Autodesk Fusion 360 part; units mm, degrees
note: some values were not read from the file. Chosen so that the rebuilt part matches the saved one: which bodies a step acts on. Set by a fixed rule: which sketch regions a step uses.
(part 2 of 6)
sketch "Sketch66" plane through (0, 0, 40) normal (0, 0, 1) x (-1, 0, 0)
  line L0 (-70.6667, -24.0741) -> (-70.6667, -4)
  line L1 (-70.6667, -4) -> (-88.8889, -4)
  line L2 (-88.8889, -4) -> (-88.8889, 0)
  line L3 (-88.8889, 0) -> (-111.1111, 0)
  line L4 (-111.1111, 0) -> (-111.1111, -4)
  line L5 (-111.1111, -4) -> (-129.3333, -4)
  line L6 (-129.3333, -4) -> (-129.3333, -22.2222)
  line L7 (-129.3333, -22.2222) -> (-137.3333, -22.2222)
  line L8 (-137.3333, -22.2222) -> (-137.3333, -4)
  line L9 (-137.3333, -4) -> (-155.5556, -4)
  line L10 (-155.5556, -4) -> (-155.5556, 0)
  line L11 (-155.5556, 0) -> (-177.7778, 0)
  line L12 (-177.7778, 0) -> (-177.7778, -4)
  line L13 (-177.7778, -4) -> (-196, -4)
  line L14 (-196, -4) -> (-196, -22.2222)
  line L15 (-196, -22.2222) -> (-200, -22.2222)
  line L16 (-200, -22.2222) -> (-200, -44.4444)
  line L17 (-200, -44.4444) -> (-196, -44.4444)
  line L18 (-196, -44.4444) -> (-196, -62.6667)
  line L19 (-196, -62.6667) -> (-177.7778, -62.6667)
  line L20 (-177.7778, -62.6667) -> (-177.7778, -70.6667)
  line L21 (-177.7778, -70.6667) -> (-196, -70.6667)
  line L22 (-196, -70.6667) -> (-196, -88.8889)
  line L23 (-196, -88.8889) -> (-200, -88.8889)
  line L24 (-200, -88.8889) -> (-200, -111.1111)
  line L25 (-200, -111.1111) -> (-196, -111.1111)
  line L26 (-196, -111.1111) -> (-196, -129.3333)
  line L27 (-196, -129.3333) -> (-177.7778, -129.3333)
  line L28 (-177.7778, -129.3333) -> (-177.7778, -137.3333)
  line L29 (-177.7778, -137.3333) -> (-196, -137.3333)
  line L30 (-196, -137.3333) -> (-196, -155.5556)
  line L31 (-196, -155.5556) -> (-200, -155.5556)
  line L32 (-200, -155.5556) -> (-200, -177.7778)
  line L33 (-200, -177.7778) -> (-196, -177.7778)
  line L34 (-196, -177.7778) -> (-196, -196)
  line L35 (-196, -196) -> (-177.7778, -196)
  line L36 (-177.7778, -196) -> (-177.7778, -200)
  line L37 (-177.7778, -200) -> (-155.5556, -200)
  line L38 (-155.5556, -200) -> (-155.5556, -196)
  line L39 (-155.5556, -196) -> (-137.3333, -196)
  line L40 (-137.3333, -196) -> (-137.3333, -177.7778)
  line L41 (-137.3333, -177.7778) -> (-129.3333, -177.7778)
  line L42 (-129.3333, -177.7778) -> (-129.3333, -196)
  line L43 (-129.3333, -196) -> (-111.1111, -196)
  line L44 (-111.1111, -196) -> (-111.1111, -200)
  line L45 (-111.1111, -200) -> (-88.8889, -200)
  line L46 (-88.8889, -200) -> (-88.8889, -196)
  line L47 (-88.8889, -196) -> (-70.6667, -196)
  line L48 (-70.6667, -196) -> (-70.6667, -177.7778)
  line L49 (-70.6667, -177.7778) -> (-62.6667, -177.7778)
  line L50 (-62.6667, -177.7778) -> (-62.6667, -196)
  line L51 (-62.6667, -196) -> (-44.4444, -196)
  line L52 (-44.4444, -196) -> (-44.4444, -200)
  line L53 (-44.4444, -200) -> (-22.2222, -200)
  line L54 (-22.2222, -200) -> (-22.2222, -196)
  line L55 (-22.2222, -196) -> (-4, -196)
  line L56 (-4, -196) -> (-4, -177.7778)
  line L57 (-4, -177.7778) -> (0, -177.7778)
  line L58 (0, -177.7778) -> (0, -155.5556)
  line L59 (0, -155.5556) -> (-4, -155.5556)
  line L60 (-4, -155.5556) -> (-4, -137.3333)
  line L61 (-4, -137.3333) -> (-22.2222, -137.3333)
  line L62 (-22.2222, -137.3333) -> (-22.2222, -129.3333)
  line L63 (-22.2222, -129.3333) -> (-4, -129.3333)
  line L64 (-4, -129.3333) -> (-4, -111.1111)
  line L65 (-4, -111.1111) -> (0, -111.1111)
  line L66 (0, -111.1111) -> (0, -88.8889)
  line L67 (0, -88.8889) -> (-4, -88.8889)
  line L68 (-4, -88.8889) -> (-4, -70.6667)
  line L69 (-4, -70.6667) -> (-22.2222, -70.6667)
  line L70 (-22.2222, -70.6667) -> (-22.2222, -62.6667)
  line L71 (-22.2222, -62.6667) -> (-4, -62.6667)
  line L72 (-4, -62.6667) -> (-4, -44.4444)
  line L73 (-4, -44.4444) -> (0, -44.4444)
  line L74 (0, -44.4444) -> (0, -22.2222)
  line L75 (0, -22.2222) -> (-4, -22.2222)
  line L76 (-4, -22.2222) -> (-4, -4)
  line L77 (-4, -4) -> (-22.2222, -4)
  line L78 (-22.2222, -4) -> (-22.2222, 0)
  line L79 (-22.2222, 0) -> (-44.4444, 0)
  line L80 (-44.4444, 0) -> (-44.4444, -4)
  line L81 (-44.4444, -4) -> (-62.6667, -4)
  line L82 (-62.6667, -4) -> (-62.6667, -24.0741)
  line L83 (-62.6667, -24.0741) -> (-66.1667, -24.0741)
  line L84 (-66.1667, -24.0741) -> (-66.1667, -42.5926)
  line L85 (-66.1667, -42.5926) -> (-62.6667, -42.5926)
  line L86 (-62.6667, -42.5926) -> (-62.6667, -62.6667)
  line L87 (-62.6667, -62.6667) -> (-44.4444, -62.6667)
  line L88 (-44.4444, -62.6667) -> (-44.4444, -70.6667)
  line L89 (-44.4444, -70.6667) -> (-62.6667, -70.6667)
  line L90 (-62.6667, -70.6667) -> (-62.6667, -88.8889)
  line L91 (-62.6667, -88.8889) -> (-70.6667, -88.8889)
  line L92 (-70.6667, -88.8889) -> (-70.6667, -70.6667)
  line L93 (-70.6667, -70.6667) -> (-88.8889, -70.6667)
  line L94 (-88.8889, -70.6667) -> (-88.8889, -62.6667)
  line L95 (-88.8889, -62.6667) -> (-70.6667, -62.6667)
  line L96 (-70.6667, -62.6667) -> (-70.6667, -42.5926)
  line L97 (-70.6667, -42.5926) -> (-67.1667, -42.5926)
  line L98 (-67.1667, -42.5926) -> (-67.1667, -24.0741)
  line L99 (-67.1667, -24.0741) -> (-70.6667, -24.0741)
  line L100 (-129.3333, -70.6667) -> (-129.3333, -88.8889)
  line L101 (-129.3333, -88.8889) -> (-137.3333, -88.8889)
  line L102 (-137.3333, -88.8889) -> (-137.3333, -70.6667)
  line L103 (-137.3333, -70.6667) -> (-155.5556, -70.6667)
  line L104 (-155.5556, -70.6667) -> (-155.5556, -62.6667)
  line L105 (-155.5556, -62.6667) -> (-137.3333, -62.6667)
  line L106 (-137.3333, -62.6667) -> (-137.3333, -44.4444)
  line L107 (-137.3333, -44.4444) -> (-129.3333, -44.4444)
  line L108 (-129.3333, -44.4444) -> (-129.3333, -62.6667)
  line L109 (-129.3333, -62.6667) -> (-111.1111, -62.6667)
  line L110 (-111.1111, -62.6667) -> (-111.1111, -70.6667)
  line L111 (-111.1111, -70.6667) -> (-129.3333, -70.6667)
  line L112 (-129.3333, -137.3333) -> (-129.3333, -155.5556)
  line L113 (-129.3333, -155.5556) -> (-137.3333, -155.5556)
  line L114 (-137.3333, -155.5556) -> (-137.3333, -137.3333)
  line L115 (-137.3333, -137.3333) -> (-155.5556, -137.3333)
  line L116 (-155.5556, -137.3333) -> (-155.5556, -129.3333)
  line L117 (-155.5556, -129.3333) -> (-137.3333, -129.3333)
  line L118 (-137.3333, -129.3333) -> (-137.3333, -111.1111)
  line L119 (-137.3333, -111.1111) -> (-129.3333, -111.1111)
  line L120 (-129.3333, -111.1111) -> (-129.3333, -129.3333)
  line L121 (-129.3333, -129.3333) -> (-111.1111, -129.3333)
  line L122 (-111.1111, -129.3333) -> (-111.1111, -137.3333)
  line L123 (-111.1111, -137.3333) -> (-129.3333, -137.3333)
  line L124 (-62.6667, -137.3333) -> (-62.6667, -155.5556)
  line L125 (-62.6667, -155.5556) -> (-70.6667, -155.5556)
  line L126 (-70.6667, -155.5556) -> (-70.6667, -137.3333)
  line L127 (-70.6667, -137.3333) -> (-88.8889, -137.3333)
  line L128 (-88.8889, -137.3333) -> (-88.8889, -129.3333)
  line L129 (-88.8889, -129.3333) -> (-70.6667, -129.3333)
  line L130 (-70.6667, -129.3333) -> (-70.6667, -111.1111)
  line L131 (-70.6667, -111.1111) -> (-62.6667, -111.1111)
  line L132 (-62.6667, -111.1111) -> (-62.6667, -129.3333)
  line L133 (-62.6667, -129.3333) -> (-44.4444, -129.3333)
  line L134 (-44.4444, -129.3333) -> (-44.4444, -137.3333)
  line L135 (-44.4444, -137.3333) -> (-62.6667, -137.3333)
  line L136 (-22.2222, -70.6667) -> (-24.0741, -70.6667)
  line L137 (-24.0741, -70.6667) -> (-24.0741, -62.6667)
  line L138 (-24.0741, -62.6667) -> (-22.2222, -62.6667)
  line L139 (-22.2222, -62.6667) -> (-22.2222, -70.6667)
  line L140 (-22.2222, -67.1667) -> (-44.4444, -67.1667)
  line L141 (-44.4444, -67.1667) -> (-44.4444, -66.1667)
  line L142 (-44.4444, -66.1667) -> (-22.2222, -66.1667)
  line L143 (-22.2222, -66.1667) -> (-22.2222, -67.1667)
  line L144 (-44.4444, -70.6667) -> (-42.5926, -70.6667)
  line L145 (-42.5926, -70.6667) -> (-42.5926, -62.6667)
  line L146 (-42.5926, -62.6667) -> (-44.4444, -62.6667)
  line L147 (-44.4444, -62.6667) -> (-44.4444, -70.6667)
  line L148 (-4, -44.4444) -> (-0.5, -44.4444)
  line L149 (-0.5, -44.4444) -> (-0.5, -42.5926)
  line L150 (-0.5, -42.5926) -> (-4, -42.5926)
  line L151 (-4, -42.5926) -> (-4, -44.4444)
  line L152 (-4, -22.2222) -> (-0.5, -22.2222)
  line L153 (-0.5, -22.2222) -> (-0.5, -24.0741)
  line L154 (-0.5, -24.0741) -> (-4, -24.0741)
  line L155 (-4, -24.0741) -> (-4, -22.2222)
  line L156 (0, -44.4444) -> (-0.5, -44.4444)
  line L157 (-0.5, -44.4444) -> (-0.5, -22.2222)
  line L158 (-0.5, -22.2222) -> (0, -22.2222)
  line L159 (0, -22.2222) -> (0, -44.4444)
  line L160 (-22.2222, -4) -> (-24.0741, -4)
  line L161 (-24.0741, -4) -> (-24.0741, -0.5)
  line L162 (-24.0741, -0.5) -> (-22.2222, -0.5)
  line L163 (-22.2222, -0.5) -> (-22.2222, -4)
  line L164 (-22.2222, 0) -> (-44.4444, 0)
  line L165 (-44.4444, 0) -> (-44.4444, -0.5)
  line L166 (-44.4444, -0.5) -> (-22.2222, -0.5)
  line L167 (-22.2222, -0.5) -> (-22.2222, 0)
  line L168 (-44.4444, -4) -> (-42.5926, -4)
  line L169 (-42.5926, -4) -> (-42.5926, -0.5)
  line L170 (-42.5926, -0.5) -> (-44.4444, -0.5)
  line L171 (-44.4444, -0.5) -> (-44.4444, -4)
  dimension "d309" = 22.2222
  dimension "d310" = 1.8519
  dimension "d311" = 1.8519
  dimension "d312" = 8
  dimension "d313" = 8
  dimension "d314" = 1
  dimension "d315" = 3.5
  dimension "d319" = 0.5
  dimension "d320" = 3.5
  dimension "d321" = 1.8519
  dimension "d322" = 1.8519
  dimension "d323" = 3.5
  dimension "d324" = 22.2222
  dimension "d327" = 3.5
  dimension "d328" = 0.5
  dimension "d329" = 1.8519
  dimension "d330" = 22.2222
  dimension "d331" = 3.5
  dimension "d332" = 1.8519
  constraint horizontal L136
  constraint vertical L137
  constraint horizontal L138
  constraint vertical L139
  constraint coincident L69.end L70.start
  constraint horizontal L140
  constraint vertical L141
  constraint horizontal L142
  constraint vertical L143
  constraint coincident L70 L140.start
  constraint horizontal L144
  constraint vertical L145
  constraint horizontal L146
  constraint vertical L147
  constraint coincident L88.end L89.start
  constraint horizontal L148
  constraint vertical L149
  constraint horizontal L150
  constraint vertical L151
  constraint coincident L72.end L73.start
  constraint horizontal L152
  constraint vertical L153
  constraint horizontal L154
  constraint vertical L155
  constraint coincident L75.end L76.start
  constraint horizontal L156
  constraint vertical L157
  constraint horizontal L158
  constraint vertical L159
  constraint coincident L73.end L74.start
  constraint horizontal L160
  constraint vertical L161
  constraint horizontal L162
  constraint vertical L163
  constraint coincident L77.end L78.start
  constraint horizontal L164
  constraint vertical L165
  constraint horizontal L166
  constraint vertical L167
  constraint coincident L78.end L79.start
  constraint horizontal L168
  constraint vertical L169
  constraint horizontal L170
  constraint vertical L171
  constraint coincident L80.end L81.start
  measures "d309" distance of L141.end L142.end
  measures "d310" distance of L137.end L70.end
  measures "d311" distance of L145.end L87.end
  measures "d312" distance of L69.end L70.end
  measures "d313" distance of L88.end L87.end
  measures "d314" distance of L140.end L141.end
  measures "d315" distance of L141.end L87.end
  measures "d319" distance of L152.end L74.end
  measures "d320" distance of L75.end L152.end
  measures "d321" distance of L75.end L154.end
  measures "d322" distance of L72.end L150.end
  measures "d323" distance of L149.end L150.end
  measures "d324" distance of L73.end L74.end
  measures "d327" distance of L77.end L162.end
  measures "d328" distance of L78.end L162.end
  measures "d329" distance of L161.end L162.end
  measures "d330" distance of L78.end L79.end
  measures "d331" distance of L80.end L165.end
  measures "d332" distance of L169.end L165.end
extrude "Extrude38" cut sketch "Sketch66" against normal blind 4 contours L88 L140 L144 L145 L147 | L88 L140 L141 L142 L145 L147 | L88 L142 L145 L146 L147 | L137 L140 L142 L145 | L70 L136 L137 L139 L140 | L70 L137 L139 L140 L142 L143 | L70 L137 L138 L139 L142 | L73 L148 L149 L150 L151 L157 | L73 L74 L75 L149 L153 L156 L157 L158 L159 | L80 L166 L168 L169 L170 L171 | L78 L79 L80 L162 L164 L165 L166 L167 L170 | L75 L152 L153 L154 L155 L157 | L78 L160 L161 L162 L163 L166 bodies 13 makes body 14 at (103.7037, 102.3704, 40)
sketch "Sketch67" plane through (0, 0, 0) normal (1, 0, 0) x (0, 1, 0)
sketch "Sketch68" plane through (0, 0, 40) normal (0, 0, 1) x (-1, 0, 0)
  line L0 (-4, -70.6667) -> (-24.0741, -70.6667)
  line L1 (-24.0741, -70.6667) -> (-24.0741, -67.1667)
  line L2 (-24.0741, -67.1667) -> (-42.5926, -67.1667)
  line L3 (-42.5926, -67.1667) -> (-42.5926, -70.6667)
  line L4 (-42.5926, -70.6667) -> (-62.6667, -70.6667)
  line L5 (-62.6667, -70.6667) -> (-62.6667, -88.8889)
  line L6 (-62.6667, -88.8889) -> (-70.6667, -88.8889)
  line L7 (-70.6667, -88.8889) -> (-70.6667, -70.6667)
  line L8 (-70.6667, -70.6667) -> (-88.8889, -70.6667)
  line L9 (-88.8889, -70.6667) -> (-88.8889, -62.6667)
  line L10 (-88.8889, -62.6667) -> (-70.6667, -62.6667)
  line L11 (-70.6667, -62.6667) -> (-70.6667, -42.5926)
  line L12 (-70.6667, -42.5926) -> (-67.1667, -42.5926)
  line L13 (-67.1667, -42.5926) -> (-67.1667, -24.0741)
  line L14 (-67.1667, -24.0741) -> (-70.6667, -24.0741)
  line L15 (-70.6667, -24.0741) -> (-70.6667, -4)
  line L16 (-70.6667, -4) -> (-88.8889, -4)
  line L17 (-88.8889, -4) -> (-88.8889, 0)
  line L18 (-88.8889, 0) -> (-111.1111, 0)
  line L19 (-111.1111, 0) -> (-111.1111, -4)
  line L20 (-111.1111, -4) -> (-129.3333, -4)
  line L21 (-129.3333, -4) -> (-129.3333, -22.2222)
  line L22 (-129.3333, -22.2222) -> (-137.3333, -22.2222)
  line L23 (-137.3333, -22.2222) -> (-137.3333, -4)
  line L24 (-137.3333, -4) -> (-155.5556, -4)
  line L25 (-155.5556, -4) -> (-155.5556, 0)
  line L26 (-155.5556, 0) -> (-177.7778, 0)
  line L27 (-177.7778, 0) -> (-177.7778, -4)
  line L28 (-177.7778, -4) -> (-196, -4)
  line L29 (-196, -4) -> (-196, -22.2222)
  line L30 (-196, -22.2222) -> (-200, -22.2222)
  line L31 (-200, -22.2222) -> (-200, -44.4444)
  line L32 (-200, -44.4444) -> (-196, -44.4444)
  line L33 (-196, -44.4444) -> (-196, -62.6667)
  line L34 (-196, -62.6667) -> (-177.7778, -62.6667)
  line L35 (-177.7778, -62.6667) -> (-177.7778, -70.6667)
  line L36 (-177.7778, -70.6667) -> (-196, -70.6667)
  line L37 (-196, -70.6667) -> (-196, -88.8889)
  line L38 (-196, -88.8889) -> (-200, -88.8889)
  line L39 (-200, -88.8889) -> (-200, -111.1111)
  line L40 (-200, -111.1111) -> (-196, -111.1111)
  line L41 (-196, -111.1111) -> (-196, -129.3333)
  line L42 (-196, -129.3333) -> (-177.7778, -129.3333)
  line L43 (-177.7778, -129.3333) -> (-177.7778, -137.3333)
  line L44 (-177.7778, -137.3333) -> (-196, -137.3333)
  line L45 (-196, -137.3333) -> (-196, -155.5556)
  line L46 (-196, -155.5556) -> (-200, -155.5556)
  line L47 (-200, -155.5556) -> (-200, -177.7778)
  line L48 (-200, -177.7778) -> (-196, -177.7778)
  line L49 (-196, -177.7778) -> (-196, -196)
  line L50 (-196, -196) -> (-177.7778, -196)
  line L51 (-177.7778, -196) -> (-177.7778, -200)
  line L52 (-177.7778, -200) -> (-155.5556, -200)
  line L53 (-155.5556, -200) -> (-155.5556, -196)
  line L54 (-155.5556, -196) -> (-137.3333, -196)
  line L55 (-137.3333, -196) -> (-137.3333, -177.7778)
  line L56 (-137.3333, -177.7778) -> (-129.3333, -177.7778)
  line L57 (-129.3333, -177.7778) -> (-129.3333, -196)
  line L58 (-129.3333, -196) -> (-111.1111, -196)
  line L59 (-111.1111, -196) -> (-111.1111, -200)
  line L60 (-111.1111, -200) -> (-88.8889, -200)
  line L61 (-88.8889, -200) -> (-88.8889, -196)
  line L62 (-88.8889, -196) -> (-70.6667, -196)
  line L63 (-70.6667, -196) -> (-70.6667, -177.7778)
  line L64 (-70.6667, -177.7778) -> (-62.6667, -177.7778)
  line L65 (-62.6667, -177.7778) -> (-62.6667, -196)
  line L66 (-62.6667, -196) -> (-44.4444, -196)
  line L67 (-44.4444, -196) -> (-44.4444, -200)
  line L68 (-44.4444, -200) -> (-22.2222, -200)
  line L69 (-22.2222, -200) -> (-22.2222, -196)
  line L70 (-22.2222, -196) -> (-4, -196)
  line L71 (-4, -196) -> (-4, -177.7778)
  line L72 (-4, -177.7778) -> (0, -177.7778)
  line L73 (0, -177.7778) -> (0, -155.5556)
  line L74 (0, -155.5556) -> (-4, -155.5556)
  line L75 (-4, -155.5556) -> (-4, -137.3333)
  line L76 (-4, -137.3333) -> (-22.2222, -137.3333)
  line L77 (-22.2222, -137.3333) -> (-22.2222, -129.3333)
  line L78 (-22.2222, -129.3333) -> (-4, -129.3333)
  line L79 (-4, -129.3333) -> (-4, -111.1111)
  line L80 (-4, -111.1111) -> (0, -111.1111)
  line L81 (0, -111.1111) -> (0, -88.8889)
  line L82 (0, -88.8889) -> (-4, -88.8889)
  line L83 (-4, -88.8889) -> (-4, -70.6667)
  line L84 (-129.3333, -70.6667) -> (-129.3333, -88.8889)
  line L85 (-129.3333, -88.8889) -> (-137.3333, -88.8889)
  line L86 (-137.3333, -88.8889) -> (-137.3333, -70.6667)
  line L87 (-137.3333, -70.6667) -> (-155.5556, -70.6667)
  line L88 (-155.5556, -70.6667) -> (-155.5556, -62.6667)
  line L89 (-155.5556, -62.6667) -> (-137.3333, -62.6667)
  line L90 (-137.3333, -62.6667) -> (-137.3333, -44.4444)
  line L91 (-137.3333, -44.4444) -> (-129.3333, -44.4444)
  line L92 (-129.3333, -44.4444) -> (-129.3333, -62.6667)
  line L93 (-129.3333, -62.6667) -> (-111.1111, -62.6667)
  line L94 (-111.1111, -62.6667) -> (-111.1111, -70.6667)
  line L95 (-111.1111, -70.6667) -> (-129.3333, -70.6667)
  line L96 (-129.3333, -137.3333) -> (-129.3333, -155.5556)
  line L97 (-129.3333, -155.5556) -> (-137.3333, -155.5556)
  line L98 (-137.3333, -155.5556) -> (-137.3333, -137.3333)
  line L99 (-137.3333, -137.3333) -> (-155.5556, -137.3333)
  line L100 (-155.5556, -137.3333) -> (-155.5556, -129.3333)
  line L101 (-155.5556, -129.3333) -> (-137.3333, -129.3333)
  line L102 (-137.3333, -129.3333) -> (-137.3333, -111.1111)
  line L103 (-137.3333, -111.1111) -> (-129.3333, -111.1111)
  line L104 (-129.3333, -111.1111) -> (-129.3333, -129.3333)
  line L105 (-129.3333, -129.3333) -> (-111.1111, -129.3333)
  line L106 (-111.1111, -129.3333) -> (-111.1111, -137.3333)
  line L107 (-111.1111, -137.3333) -> (-129.3333, -137.3333)
  line L108 (-62.6667, -137.3333) -> (-62.6667, -155.5556)
  line L109 (-62.6667, -155.5556) -> (-70.6667, -155.5556)
  line L110 (-70.6667, -155.5556) -> (-70.6667, -137.3333)
  line L111 (-70.6667, -137.3333) -> (-88.8889, -137.3333)
  line L112 (-88.8889, -137.3333) -> (-88.8889, -129.3333)
  line L113 (-88.8889, -129.3333) -> (-70.6667, -129.3333)
  line L114 (-70.6667, -129.3333) -> (-70.6667, -111.1111)
  line L115 (-70.6667, -111.1111) -> (-62.6667, -111.1111)
  line L116 (-62.6667, -111.1111) -> (-62.6667, -129.3333)
  line L117 (-62.6667, -129.3333) -> (-44.4444, -129.3333)
  line L118 (-44.4444, -129.3333) -> (-44.4444, -137.3333)
  line L119 (-44.4444, -137.3333) -> (-62.6667, -137.3333)
  line L120 (-88.8889, -4) -> (-90.7407, -4)
  line L121 (-90.7407, -4) -> (-90.7407, -0.5)
  line L122 (-90.7407, -0.5) -> (-88.8889, -0.5)
  line L123 (-88.8889, -0.5) -> (-88.8889, -4)
  line L124 (-88.8889, 0) -> (-111.1111, 0)
  line L125 (-111.1111, 0) -> (-111.1111, -0.5)
  line L126 (-111.1111, -0.5) -> (-88.8889, -0.5)
  line L127 (-88.8889, -0.5) -> (-88.8889, 0)
  line L128 (-111.1111, -4) -> (-109.2593, -4)
  line L129 (-109.2593, -4) -> (-109.2593, -0.5)
  line L130 (-109.2593, -0.5) -> (-111.1111, -0.5)
  line L131 (-111.1111, -0.5) -> (-111.1111, -4)
  line L132 (-129.3333, -44.4444) -> (-137.3333, -44.4444)
  line L133 (-137.3333, -44.4444) -> (-137.3333, -42.5926)
  line L134 (-137.3333, -42.5926) -> (-129.3333, -42.5926)
  line L135 (-129.3333, -42.5926) -> (-129.3333, -44.4444)
  line L136 (-132.8333, -44.4444) -> (-133.8333, -44.4444)
  line L137 (-133.8333, -44.4444) -> (-133.8333, -22.2222)
  line L138 (-133.8333, -22.2222) -> (-132.8333, -22.2222)
  line L139 (-132.8333, -22.2222) -> (-132.8333, -44.4444)
  line L140 (-129.3333, -22.2222) -> (-137.3333, -22.2222)
  line L141 (-137.3333, -22.2222) -> (-137.3333, -24.0741)
  line L142 (-137.3333, -24.0741) -> (-129.3333, -24.0741)
  line L143 (-129.3333, -24.0741) -> (-129.3333, -22.2222)
  line L144 (-88.8889, -70.6667) -> (-90.7407, -70.6667)
  line L145 (-90.7407, -70.6667) -> (-90.7407, -62.6667)
  line L146 (-90.7407, -62.6667) -> (-88.8889, -62.6667)
  line L147 (-88.8889, -62.6667) -> (-88.8889, -70.6667)
  line L148 (-111.1111, -70.6667) -> (-109.2593, -70.6667)
  line L149 (-109.2593, -70.6667) -> (-109.2593, -62.6667)
  line L150 (-109.2593, -62.6667) -> (-111.1111, -62.6667)
  line L151 (-111.1111, -62.6667) -> (-111.1111, -70.6667)
  line L152 (-88.8889, -67.1667) -> (-111.1111, -67.1667)
  line L153 (-111.1111, -67.1667) -> (-111.1111, -66.1667)
  line L154 (-111.1111, -66.1667) -> (-88.8889, -66.1667)
  line L155 (-88.8889, -66.1667) -> (-88.8889, -67.1667)
  dimension "d335" = 0.5
  dimension "d337" = 3.5
  dimension "d338" = 1.8519
  dimension "d339" = 22.2222
  dimension "d340" = 1.8519
  dimension "d341" = 3.5
  dimension "d342" = 1.8519
  dimension "d343" = 8
  dimension "d344" = 22.2222
  dimension "d345" = 1
  dimension "d346" = 3.5
  dimension "d347" = 1.8519
  dimension "d348" = 8
  dimension "d349" = 1.8519
  dimension "d350" = 8
  dimension "d351" = 1
  dimension "d352" = 22.2222
  dimension "d353" = 3.5
  dimension "d354" = 1.8519
  dimension "d355" = 8
  dimension "d356" = 3.5
  constraint horizontal L120
  constraint vertical L121
  constraint horizontal L122
  constraint vertical L123
  constraint coincident L16.end L17.start
  constraint horizontal L124
  constraint vertical L125
  constraint horizontal L126
  constraint vertical L127
  constraint coincident L17.end L18.start
  constraint horizontal L128
  constraint vertical L129
  constraint horizontal L130
  constraint vertical L131
  constraint coincident L19.end L20.start
  constraint horizontal L132
  constraint vertical L133
  constraint horizontal L134
  constraint vertical L135
  constraint coincident L91.end L92.start
  constraint horizontal L136
  constraint vertical L137
  constraint horizontal L138
  constraint vertical L139
  constraint coincident L91 L136.start
  constraint horizontal L140
  constraint vertical L141
  constraint horizontal L142
  constraint vertical L143
  constraint coincident L21.end L22.start
  constraint horizontal L144
  constraint vertical L145
  constraint horizontal L146
  constraint vertical L147
  constraint coincident L8.end L9.start
  constraint horizontal L148
  constraint vertical L149
  constraint horizontal L150
  constraint vertical L151
  constraint coincident L94.end L95.start
  constraint horizontal L152
  constraint vertical L153
  constraint horizontal L154
  constraint vertical L155
  constraint coincident L147 L152.start
  measures "d335" distance of L17.end L122.end
  measures "d337" distance of L16.end L122.end
  measures "d338" distance of L121.end L122.end
  measures "d339" distance of L17.end L18.end
  measures "d340" distance of L129.end L125.end
  measures "d341" distance of L19.end L125.end
  measures "d342" distance of L22.end L141.end
  measures "d343" distance of L21.end L22.end
  measures "d344" distance of L136.end L137.end
  measures "d345" distance of L137.end L138.end
  measures "d346" distance of L22.end L137.end
  measures "d347" distance of L90.end L133.end
  measures "d348" distance of L133.end L134.end
  measures "d349" distance of L149.end L93.end
  measures "d350" distance of L94.end L93.end
  measures "d351" distance of L152.end L153.end
  measures "d352" distance of L153.end L154.end
  measures "d353" distance of L93.end L153.end
  measures "d354" distance of L8.end L144.end
  measures "d355" distance of L144.end L145.end
  measures "d356" distance of L9.end L154.end
extrude "Extrude39" cut sketch "Sketch68" against normal blind 4 contours L9 L144 L145 L147 L152 | L9 L145 L147 L152 L154 L155 | L9 L145 L146 L147 L154 | L145 L149 L152 L154 | L94 L149 L151 L152 L153 L154 | L94 L148 L149 L151 L152 | L94 L149 L150 L151 L154 | L91 L132 L134 L135 L139 | L91 L132 L134 L136 L137 L139 | L17 L120 L121 L122 L123 L126 | L91 L132 L133 L134 L137 | L134 L137 L139 L142 | L17 L18 L19 L122 L124 L125 L126 L127 L130 | L22 L137 L138 L139 L140 L142 | L22 L139 L140 L142 L143 | L22 L137 L140 L141 L142 | L19 L126 L128 L129 L130 L131 bodies 14 makes body 15 at (103.7037, 169.037, 40)
sketch "Sketch71" plane through (0, 0, 40) normal (0, 0, 1) x (-1, 0, 0)
  line L0 (-109.2593, -70.6667) -> (-129.3333, -70.6667)
  line L1 (-129.3333, -70.6667) -> (-129.3333, -88.8889)
  line L2 (-129.3333, -88.8889) -> (-137.3333, -88.8889)
  line L3 (-137.3333, -88.8889) -> (-137.3333, -70.6667)
  line L4 (-137.3333, -70.6667) -> (-155.5556, -70.6667)
  line L5 (-155.5556, -70.6667) -> (-155.5556, -62.6667)
  line L6 (-155.5556, -62.6667) -> (-137.3333, -62.6667)
  line L7 (-137.3333, -62.6667) -> (-137.3333, -42.5926)
  line L8 (-137.3333, -42.5926) -> (-133.8333, -42.5926)
  line L9 (-133.8333, -42.5926) -> (-133.8333, -24.0741)
  line L10 (-133.8333, -24.0741) -> (-137.3333, -24.0741)
  line L11 (-137.3333, -24.0741) -> (-137.3333, -4)
  line L12 (-137.3333, -4) -> (-155.5556, -4)
  line L13 (-155.5556, -4) -> (-155.5556, 0)
  line L14 (-155.5556, 0) -> (-177.7778, 0)
  line L15 (-177.7778, 0) -> (-177.7778, -4)
  line L16 (-177.7778, -4) -> (-196, -4)
  line L17 (-196, -4) -> (-196, -22.2222)
  line L18 (-196, -22.2222) -> (-200, -22.2222)
  line L19 (-200, -22.2222) -> (-200, -44.4444)
  line L20 (-200, -44.4444) -> (-196, -44.4444)
  line L21 (-196, -44.4444) -> (-196, -62.6667)
  line L22 (-196, -62.6667) -> (-177.7778, -62.6667)
  line L23 (-177.7778, -62.6667) -> (-177.7778, -70.6667)
  line L24 (-177.7778, -70.6667) -> (-196, -70.6667)
  line L25 (-196, -70.6667) -> (-196, -88.8889)
  line L26 (-196, -88.8889) -> (-200, -88.8889)
  line L27 (-200, -88.8889) -> (-200, -111.1111)
  line L28 (-200, -111.1111) -> (-196, -111.1111)
  line L29 (-196, -111.1111) -> (-196, -129.3333)
  line L30 (-196, -129.3333) -> (-177.7778, -129.3333)
  line L31 (-177.7778, -129.3333) -> (-177.7778, -137.3333)
  line L32 (-177.7778, -137.3333) -> (-196, -137.3333)
  line L33 (-196, -137.3333) -> (-196, -155.5556)
  line L34 (-196, -155.5556) -> (-200, -155.5556)
  line L35 (-200, -155.5556) -> (-200, -177.7778)
  line L36 (-200, -177.7778) -> (-196, -177.7778)
  line L37 (-196, -177.7778) -> (-196, -196)
  line L38 (-196, -196) -> (-177.7778, -196)
  line L39 (-177.7778, -196) -> (-177.7778, -200)
  line L40 (-177.7778, -200) -> (-155.5556, -200)
  line L41 (-155.5556, -200) -> (-155.5556, -196)
  line L42 (-155.5556, -196) -> (-137.3333, -196)
  line L43 (-137.3333, -196) -> (-137.3333, -177.7778)
  line L44 (-137.3333, -177.7778) -> (-129.3333, -177.7778)
  line L45 (-129.3333, -177.7778) -> (-129.3333, -196)
  line L46 (-129.3333, -196) -> (-111.1111, -196)
  line L47 (-111.1111, -196) -> (-111.1111, -200)
  line L48 (-111.1111, -200) -> (-88.8889, -200)
  line L49 (-88.8889, -200) -> (-88.8889, -196)
  line L50 (-88.8889, -196) -> (-70.6667, -196)
  line L51 (-70.6667, -196) -> (-70.6667, -177.7778)
  line L52 (-70.6667, -177.7778) -> (-62.6667, -177.7778)
  line L53 (-62.6667, -177.7778) -> (-62.6667, -196)
  line L54 (-62.6667, -196) -> (-44.4444, -196)
  line L55 (-44.4444, -196) -> (-44.4444, -200)
  line L56 (-44.4444, -200) -> (-22.2222, -200)
  line L57 (-22.2222, -200) -> (-22.2222, -196)
  line L58 (-22.2222, -196) -> (-4, -196)
  line L59 (-4, -196) -> (-4, -177.7778)
  line L60 (-4, -177.7778) -> (0, -177.7778)
  line L61 (0, -177.7778) -> (0, -155.5556)
  line L62 (0, -155.5556) -> (-4, -155.5556)
  line L63 (-4, -155.5556) -> (-4, -137.3333)
  line L64 (-4, -137.3333) -> (-22.2222, -137.3333)
  line L65 (-22.2222, -137.3333) -> (-22.2222, -129.3333)
  line L66 (-22.2222, -129.3333) -> (-4, -129.3333)
  line L67 (-4, -129.3333) -> (-4, -111.1111)
  line L68 (-4, -111.1111) -> (0, -111.1111)
  line L69 (0, -111.1111) -> (0, -88.8889)
  line L70 (0, -88.8889) -> (-4, -88.8889)
  line L71 (-4, -88.8889) -> (-4, -70.6667)
  line L72 (-4, -70.6667) -> (-24.0741, -70.6667)
  line L73 (-24.0741, -70.6667) -> (-24.0741, -67.1667)
  line L74 (-24.0741, -67.1667) -> (-42.5926, -67.1667)
  line L75 (-42.5926, -67.1667) -> (-42.5926, -70.6667)
  line L76 (-42.5926, -70.6667) -> (-62.6667, -70.6667)
  line L77 (-62.6667, -70.6667) -> (-62.6667, -88.8889)
  line L78 (-62.6667, -88.8889) -> (-70.6667, -88.8889)
  line L79 (-70.6667, -88.8889) -> (-70.6667, -70.6667)
  line L80 (-70.6667, -70.6667) -> (-90.7407, -70.6667)
  line L81 (-90.7407, -70.6667) -> (-90.7407, -67.1667)
  line L82 (-90.7407, -67.1667) -> (-109.2593, -67.1667)
  line L83 (-109.2593, -67.1667) -> (-109.2593, -70.6667)
  line L84 (-129.3333, -137.3333) -> (-129.3333, -155.5556)
  line L85 (-129.3333, -155.5556) -> (-137.3333, -155.5556)
  line L86 (-137.3333, -155.5556) -> (-137.3333, -137.3333)
  line L87 (-137.3333, -137.3333) -> (-155.5556, -137.3333)
  line L88 (-155.5556, -137.3333) -> (-155.5556, -129.3333)
  line L89 (-155.5556, -129.3333) -> (-137.3333, -129.3333)
  line L90 (-137.3333, -129.3333) -> (-137.3333, -111.1111)
  line L91 (-137.3333, -111.1111) -> (-129.3333, -111.1111)
  line L92 (-129.3333, -111.1111) -> (-129.3333, -129.3333)
  line L93 (-129.3333, -129.3333) -> (-111.1111, -129.3333)
  line L94 (-111.1111, -129.3333) -> (-111.1111, -137.3333)
  line L95 (-111.1111, -137.3333) -> (-129.3333, -137.3333)
  line L96 (-62.6667, -137.3333) -> (-62.6667, -155.5556)
  line L97 (-62.6667, -155.5556) -> (-70.6667, -155.5556)
  line L98 (-70.6667, -155.5556) -> (-70.6667, -137.3333)
  line L99 (-70.6667, -137.3333) -> (-88.8889, -137.3333)
  line L100 (-88.8889, -137.3333) -> (-88.8889, -129.3333)
  line L101 (-88.8889, -129.3333) -> (-70.6667, -129.3333)
  line L102 (-70.6667, -129.3333) -> (-70.6667, -111.1111)
  line L103 (-70.6667, -111.1111) -> (-62.6667, -111.1111)
  line L104 (-62.6667, -111.1111) -> (-62.6667, -129.3333)
  line L105 (-62.6667, -129.3333) -> (-44.4444, -129.3333)
  line L106 (-44.4444, -129.3333) -> (-44.4444, -137.3333)
  line L107 (-44.4444, -137.3333) -> (-62.6667, -137.3333)
  line L108 (-155.5556, -4) -> (-157.4074, -4)
  line L109 (-157.4074, -4) -> (-157.4074, -0.5)
  line L110 (-157.4074, -0.5) -> (-155.5556, -0.5)
  line L111 (-155.5556, -0.5) -> (-155.5556, -4)
  line L112 (-177.7778, -4) -> (-175.9259, -4)
  line L113 (-175.9259, -4) -> (-175.9259, -0.5)
  line L114 (-175.9259, -0.5) -> (-177.7778, -0.5)
  line L115 (-177.7778, -0.5) -> (-177.7778, -4)
  line L116 (-155.5556, 0) -> (-177.7778, 0)
  line L117 (-177.7778, 0) -> (-177.7778, -0.5)
  line L118 (-177.7778, -0.5) -> (-155.5556, -0.5)
  line L119 (-155.5556, -0.5) -> (-155.5556, 0)
  line L120 (-196, -44.4444) -> (-199.5, -44.4444)
  line L121 (-199.5, -44.4444) -> (-199.5, -42.5926)
  line L122 (-199.5, -42.5926) -> (-196, -42.5926)
  line L123 (-196, -42.5926) -> (-196, -44.4444)
  line L124 (-196, -22.2222) -> (-199.5, -22.2222)
  line L125 (-199.5, -22.2222) -> (-199.5, -24.0741)
  line L126 (-199.5, -24.0741) -> (-196, -24.0741)
  line L127 (-196, -24.0741) -> (-196, -22.2222)
  line L128 (-200, -22.2222) -> (-199.5, -22.2222)
  line L129 (-199.5, -22.2222) -> (-199.5, -44.4444)
  line L130 (-199.5, -44.4444) -> (-200, -44.4444)
  line L131 (-200, -44.4444) -> (-200, -22.2222)
  line L132 (-155.5556, -62.6667) -> (-157.4074, -62.6667)
  line L133 (-157.4074, -62.6667) -> (-157.4074, -70.6667)
  line L134 (-157.4074, -70.6667) -> (-155.5556, -70.6667)
  line L135 (-155.5556, -70.6667) -> (-155.5556, -62.6667)
  line L136 (-177.7778, -62.6667) -> (-175.9259, -62.6667)
  line L137 (-175.9259, -62.6667) -> (-175.9259, -70.6667)
  line L138 (-175.9259, -70.6667) -> (-177.7778, -70.6667)
  line L139 (-177.7778, -70.6667) -> (-177.7778, -62.6667)
  line L140 (-155.5556, -67.1667) -> (-177.7778, -67.1667)
  line L141 (-177.7778, -67.1667) -> (-177.7778, -66.1667)
  line L142 (-177.7778, -66.1667) -> (-155.5556, -66.1667)
  line L143 (-155.5556, -66.1667) -> (-155.5556, -67.1667)
  dimension "d363" = 3.5
  dimension "d364" = 0.5
  dimension "d365" = 22.2222
  dimension "d366" = 1.8519
  dimension "d367" = 1.8519
  dimension "d368" = 3.5
  dimension "d369" = 3.5
  dimension "d370" = 0.5
  dimension "d371" = 1.8519
  dimension "d372" = 22.2222
  dimension "d373" = 3.5
  dimension "d374" = 1.8519
  dimension "d375" = 1.8519
  dimension "d376" = 1.8519
  dimension "d377" = 8
  dimension "d378" = 8
  dimension "d379" = 1
  dimension "d380" = 3.5
  dimension "d381" = 22.2222
  constraint horizontal L108
  constraint vertical L109
  constraint horizontal L110
  constraint vertical L111
  constraint coincident L12.end L13.start
  constraint horizontal L112
  constraint vertical L113
  constraint horizontal L114
  constraint vertical L115
  constraint coincident L15.end L16.start
  constraint horizontal L116
  constraint vertical L117
  constraint horizontal L118
  constraint vertical L119
  constraint coincident L13.end L14.start
  constraint horizontal L120
  constraint vertical L121
  constraint horizontal L122
  constraint vertical L123
  constraint coincident L20.end L21.start
  constraint horizontal L124
  constraint vertical L125
  constraint horizontal L126
  constraint vertical L127
  constraint coincident L17.end L18.start
  constraint horizontal L128
  constraint vertical L129
  constraint horizontal L130
  constraint vertical L131
  constraint coincident L18.end L19.start
  constraint horizontal L132
  constraint vertical L133
  constraint horizontal L134
  constraint vertical L135
  constraint coincident L5.end L6.start
  constraint horizontal L136
  constraint vertical L137
  constraint horizontal L138
  constraint vertical L139
  constraint coincident L22.end L23.start
  constraint horizontal L140
  constraint vertical L141
  constraint horizontal L142
  constraint vertical L143
  constraint coincident L135 L140.start
  measures "d363" distance of L15.end L114.end
  measures "d364" distance of L14.end L114.end
  measures "d365" distance of L13.end L14.end
  measures "d366" distance of L109.end L110.end
  measures "d367" distance of L15.end L112.end
  measures "d368" distance of L12.end L110.end
  measures "d369" distance of L17.end L124.end
  measures "d370" distance of L18.end L124.end
  measures "d371" distance of L17.end L126.end
  measures "d372" distance of L18.end L19.end
  measures "d373" distance of L20.end L120.end
  measures "d374" distance of L20.end L122.end
  measures "d375" distance of L5.end L132.end
  measures "d376" distance of L22.end L136.end
  measures "d377" distance of L136.end L137.end
  measures "d378" distance of L5.end L4.end
  measures "d379" distance of L140.end L141.end
  measures "d380" distance of L4.end L140.start
  measures "d381" distance of L141.end L142.end
extrude "Extrude40" cut sketch "Sketch71" against normal blind 4 contours L5 L133 L134 L135 L140 | L5 L133 L135 L140 L142 L143 | L5 L132 L133 L135 L142 | L133 L137 L140 L142 | L23 L137 L139 L140 L141 L142 | L23 L137 L138 L139 L140 | L23 L136 L137 L139 L142 | L20 L120 L121 L122 L123 L129 | L18 L19 L20 L121 L125 L128 L129 L130 L131 | L13 L108 L109 L110 L111 L118 | L13 L14 L15 L110 L114 L116 L117 L118 L119 | L18 L124 L125 L126 L127 L129 | L15 L112 L113 L114 L115 L118 bodies 15 makes body 16 at (96.2963, 169.037, 40)
sketch "Sketch72" plane through (0, 0, 40) normal (0, 0, 1) x (-1, 0, 0)
  line L0 (-175.9259, -70.6667) -> (-196, -70.6667)
  line L1 (-196, -70.6667) -> (-196, -88.8889)
  line L2 (-196, -88.8889) -> (-200, -88.8889)
  line L3 (-200, -88.8889) -> (-200, -111.1111)
  line L4 (-200, -111.1111) -> (-196, -111.1111)
  line L5 (-196, -111.1111) -> (-196, -129.3333)
  line L6 (-196, -129.3333) -> (-177.7778, -129.3333)
  line L7 (-177.7778, -129.3333) -> (-177.7778, -137.3333)
  line L8 (-177.7778, -137.3333) -> (-196, -137.3333)
  line L9 (-196, -137.3333) -> (-196, -155.5556)
  line L10 (-196, -155.5556) -> (-200, -155.5556)
  line L11 (-200, -155.5556) -> (-200, -177.7778)
  line L12 (-200, -177.7778) -> (-196, -177.7778)
  line L13 (-196, -177.7778) -> (-196, -196)
  line L14 (-196, -196) -> (-177.7778, -196)
  line L15 (-177.7778, -196) -> (-177.7778, -200)
  line L16 (-177.7778, -200) -> (-155.5556, -200)
  line L17 (-155.5556, -200) -> (-155.5556, -196)
  line L18 (-155.5556, -196) -> (-137.3333, -196)
  line L19 (-137.3333, -196) -> (-137.3333, -177.7778)
  line L20 (-137.3333, -177.7778) -> (-129.3333, -177.7778)
  line L21 (-129.3333, -177.7778) -> (-129.3333, -196)
  line L22 (-129.3333, -196) -> (-111.1111, -196)
  line L23 (-111.1111, -196) -> (-111.1111, -200)
  line L24 (-111.1111, -200) -> (-88.8889, -200)
  line L25 (-88.8889, -200) -> (-88.8889, -196)
  line L26 (-88.8889, -196) -> (-70.6667, -196)
  line L27 (-70.6667, -196) -> (-70.6667, -177.7778)
  line L28 (-70.6667, -177.7778) -> (-62.6667, -177.7778)
  line L29 (-62.6667, -177.7778) -> (-62.6667, -196)
  line L30 (-62.6667, -196) -> (-44.4444, -196)
  line L31 (-44.4444, -196) -> (-44.4444, -200)
  line L32 (-44.4444, -200) -> (-22.2222, -200)
  line L33 (-22.2222, -200) -> (-22.2222, -196)
  line L34 (-22.2222, -196) -> (-4, -196)
  line L35 (-4, -196) -> (-4, -177.7778)
  line L36 (-4, -177.7778) -> (0, -177.7778)
  line L37 (0, -177.7778) -> (0, -155.5556)
  line L38 (0, -155.5556) -> (-4, -155.5556)
  line L39 (-4, -155.5556) -> (-4, -137.3333)
  line L40 (-4, -137.3333) -> (-22.2222, -137.3333)
  line L41 (-22.2222, -137.3333) -> (-22.2222, -129.3333)
  line L42 (-22.2222, -129.3333) -> (-4, -129.3333)
  line L43 (-4, -129.3333) -> (-4, -111.1111)
  line L44 (-4, -111.1111) -> (0, -111.1111)
  line L45 (0, -111.1111) -> (0, -88.8889)
  line L46 (0, -88.8889) -> (-4, -88.8889)
  line L47 (-4, -88.8889) -> (-4, -70.6667)
  line L48 (-4, -70.6667) -> (-24.0741, -70.6667)
  line L49 (-24.0741, -70.6667) -> (-24.0741, -67.1667)
  line L50 (-24.0741, -67.1667) -> (-42.5926, -67.1667)
  line L51 (-42.5926, -67.1667) -> (-42.5926, -70.6667)
  line L52 (-42.5926, -70.6667) -> (-62.6667, -70.6667)
  line L53 (-62.6667, -70.6667) -> (-62.6667, -88.8889)
  line L54 (-62.6667, -88.8889) -> (-70.6667, -88.8889)
  line L55 (-70.6667, -88.8889) -> (-70.6667, -70.6667)
  line L56 (-70.6667, -70.6667) -> (-90.7407, -70.6667)
  line L57 (-90.7407, -70.6667) -> (-90.7407, -67.1667)
  line L58 (-90.7407, -67.1667) -> (-109.2593, -67.1667)
  line L59 (-109.2593, -67.1667) -> (-109.2593, -70.6667)
  line L60 (-109.2593, -70.6667) -> (-129.3333, -70.6667)
  line L61 (-129.3333, -70.6667) -> (-129.3333, -88.8889)
  line L62 (-129.3333, -88.8889) -> (-137.3333, -88.8889)
  line L63 (-137.3333, -88.8889) -> (-137.3333, -70.6667)
  line L64 (-137.3333, -70.6667) -> (-157.4074, -70.6667)
  line L65 (-157.4074, -70.6667) -> (-157.4074, -67.1667)
  line L66 (-157.4074, -67.1667) -> (-175.9259, -67.1667)
  line L67 (-175.9259, -67.1667) -> (-175.9259, -70.6667)
  line L68 (-129.3333, -137.3333) -> (-129.3333, -155.5556)
  line L69 (-129.3333, -155.5556) -> (-137.3333, -155.5556)
  line L70 (-137.3333, -155.5556) -> (-137.3333, -137.3333)
  line L71 (-137.3333, -137.3333) -> (-155.5556, -137.3333)
  line L72 (-155.5556, -137.3333) -> (-155.5556, -129.3333)
  line L73 (-155.5556, -129.3333) -> (-137.3333, -129.3333)
  line L74 (-137.3333, -129.3333) -> (-137.3333, -111.1111)
  line L75 (-137.3333, -111.1111) -> (-129.3333, -111.1111)
  line L76 (-129.3333, -111.1111) -> (-129.3333, -129.3333)
  line L77 (-129.3333, -129.3333) -> (-111.1111, -129.3333)
  line L78 (-111.1111, -129.3333) -> (-111.1111, -137.3333)
  line L79 (-111.1111, -137.3333) -> (-129.3333, -137.3333)
  line L80 (-62.6667, -137.3333) -> (-62.6667, -155.5556)
  line L81 (-62.6667, -155.5556) -> (-70.6667, -155.5556)
  line L82 (-70.6667, -155.5556) -> (-70.6667, -137.3333)
  line L83 (-70.6667, -137.3333) -> (-88.8889, -137.3333)
  line L84 (-88.8889, -137.3333) -> (-88.8889, -129.3333)
  line L85 (-88.8889, -129.3333) -> (-70.6667, -129.3333)
  line L86 (-70.6667, -129.3333) -> (-70.6667, -111.1111)
  line L87 (-70.6667, -111.1111) -> (-62.6667, -111.1111)
  line L88 (-62.6667, -111.1111) -> (-62.6667, -129.3333)
  line L89 (-62.6667, -129.3333) -> (-44.4444, -129.3333)
  line L90 (-44.4444, -129.3333) -> (-44.4444, -137.3333)
  line L91 (-44.4444, -137.3333) -> (-62.6667, -137.3333)
  line L92 (-22.2222, -137.3333) -> (-24.0741, -137.3333)
  line L93 (-24.0741, -137.3333) -> (-24.0741, -129.3333)
  line L94 (-24.0741, -129.3333) -> (-22.2222, -129.3333)
  line L95 (-22.2222, -129.3333) -> (-22.2222, -137.3333)
  line L96 (-44.4444, -137.3333) -> (-42.5926, -137.3333)
  line L97 (-42.5926, -137.3333) -> (-42.5926, -129.3333)
  line L98 (-42.5926, -129.3333) -> (-44.4444, -129.3333)
  line L99 (-44.4444, -129.3333) -> (-44.4444, -137.3333)
  line L100 (-22.2222, -133.8333) -> (-44.4444, -133.8333)
  line L101 (-44.4444, -133.8333) -> (-44.4444, -132.8333)
  line L102 (-44.4444, -132.8333) -> (-22.2222, -132.8333)
  line L103 (-22.2222, -132.8333) -> (-22.2222, -133.8333)
  line L104 (-4, -111.1111) -> (-0.5, -111.1111)
  line L105 (-0.5, -111.1111) -> (-0.5, -109.2593)
  line L106 (-0.5, -109.2593) -> (-4, -109.2593)
  line L107 (-4, -109.2593) -> (-4, -111.1111)
  line L108 (-4, -88.8889) -> (-0.5, -88.8889)
  line L109 (-0.5, -88.8889) -> (-0.5, -90.7407)
  line L110 (-0.5, -90.7407) -> (-4, -90.7407)
  line L111 (-4, -90.7407) -> (-4, -88.8889)
  line L112 (0, -111.1111) -> (-0.5, -111.1111)
  line L113 (-0.5, -111.1111) -> (-0.5, -88.8889)
  line L114 (-0.5, -88.8889) -> (0, -88.8889)
  line L115 (0, -88.8889) -> (0, -111.1111)
  line L116 (-62.6667, -111.1111) -> (-70.6667, -111.1111)
  line L117 (-70.6667, -111.1111) -> (-70.6667, -109.2593)
  line L118 (-70.6667, -109.2593) -> (-62.6667, -109.2593)
  line L119 (-62.6667, -109.2593) -> (-62.6667, -111.1111)
  line L120 (-66.1667, -111.1111) -> (-67.1667, -111.1111)
  line L121 (-67.1667, -111.1111) -> (-67.1667, -88.8889)
  line L122 (-67.1667, -88.8889) -> (-66.1667, -88.8889)
  line L123 (-66.1667, -88.8889) -> (-66.1667, -111.1111)
  line L124 (-62.6667, -88.8889) -> (-70.6667, -88.8889)
  line L125 (-70.6667, -88.8889) -> (-70.6667, -90.7407)
  line L126 (-70.6667, -90.7407) -> (-62.6667, -90.7407)
  line L127 (-62.6667, -90.7407) -> (-62.6667, -88.8889)
  dimension "d384" = 1.8519
  dimension "d385" = 1.8519
  dimension "d386" = 8
  dimension "d387" = 8
  dimension "d388" = 1
  dimension "d389" = 3.5
  dimension "d390" = 3.5
  dimension "d391" = 1.8519
  dimension "d392" = 3.5
  dimension "d393" = 0.5
  dimension "d394" = 22.2222
  dimension "d395" = 1.8519
  dimension "d396" = 3.5
  dimension "d397" = 1.8519
  dimension "d398" = 1.8519
  dimension "d399" = 8
  dimension "d400" = 8
  dimension "d401" = 1
  dimension "d402" = 3.5
  dimension "d403" = 22.2222
  constraint horizontal L92
  constraint vertical L93
  constraint horizontal L94
  constraint vertical L95
  constraint coincident L40.end L41.start
  constraint horizontal L96
  constraint vertical L97
  constraint horizontal L98
  constraint vertical L99
  constraint coincident L90.end L91.start
  constraint horizontal L100
  constraint vertical L101
  constraint horizontal L102
  constraint vertical L103
  constraint coincident L99 L101.end
  constraint coincident L41 L100.start
  constraint horizontal L104
  constraint vertical L105
  constraint horizontal L106
  constraint vertical L107
  constraint coincident L43.end L44.start
  constraint horizontal L108
  constraint vertical L109
  constraint horizontal L110
  constraint vertical L111
  constraint coincident L46.end L47.start
  constraint horizontal L112
  constraint vertical L113
  constraint horizontal L114
  constraint vertical L115
  constraint coincident L44.end L45.start
  constraint horizontal L116
  constraint vertical L117
  constraint horizontal L118
  constraint vertical L119
  constraint coincident L87.end L88.start
  constraint horizontal L120
  constraint vertical L121
  constraint horizontal L122
  constraint vertical L123
  constraint coincident L116 L120.start
  constraint horizontal L124
  constraint vertical L125
  constraint horizontal L126
  constraint vertical L127
  constraint coincident L53.end L54.start
  measures "d384" distance of L97.end L89.end
  measures "d385" distance of L93.end L41.end
  measures "d386" distance of L40.end L41.end
  measures "d387" distance of L90.end L89.end
  measures "d388" distance of L100.start L102.end
  measures "d389" distance of L40.end L100.start
  measures "d390" distance of L89.end L101.end
  measures "d391" distance of L46.end L110.end
  measures "d392" distance of L46.end L108.end
  measures "d393" distance of L108.end L45.end
  measures "d394" distance of L44.end L45.end
  measures "d395" distance of L43.end L106.end
  measures "d396" distance of L105.end L106.end
  measures "d397" distance of L53.end L126.end
  measures "d398" distance of L87.end L118.end
  measures "d399" distance of L87.end L86.end
  measures "d400" distance of L53.end L54.end
  measures "d401" distance of L121.end L122.end
  measures "d402" distance of L86.end L120.end
  measures "d403" distance of L120.end L121.end
extrude "Extrude41" cut sketch "Sketch72" against normal blind 4 contours L54 L121 L124 L125 L126 | L54 L121 L122 L123 L124 L126 | L54 L123 L124 L126 L127 | L118 L121 L123 L126 | L87 L116 L117 L118 L121 | L87 L116 L118 L120 L121 L123 | L87 L116 L118 L119 L123 | L90 L97 L98 L99 L102 | L90 L97 L99 L100 L101 L102 | L46 L108 L109 L110 L111 L113 | L90 L96 L97 L99 L100 | L93 L97 L100 L102 | L44 L45 L46 L105 L109 L112 L113 L114 L115 | L41 L93 L95 L100 L102 L103 | L41 L93 L94 L95 L102 | L41 L92 L93 L95 L100 | L44 L104 L105 L106 L107 L113 bodies 16 makes body 17 at (96.2963, 169.037, 40)